Top Cover (Autodesk Fusion 360 design; units mm, degrees)
Autodesk Fusion 360 part; units mm, degrees
sketch "Sketch1" plane through (0, 0, 0) normal (0, 0, 1) x (1, 0, 0)
  line L0 (0, 0) -> (-187, 0)
  line L1 (-187, 0) -> (-187, 128)
  line L2 (-169, 146) -> (-18, 146)
  line L3 (0, 128) -> (0, 0)
  arc A0 (0, 128) -> (-18, 146) centre (-18, 128) ccw
  arc A1 (-169, 146) -> (-187, 128) centre (-169, 128) ccw
  line L4 (-185, 2) -> (-185, 126)
  line L5 (-2, 126) -> (-2, 2)
  line L6 (-185, 2) -> (-185, 0)
  line L7 (-2, 2) -> (-2, 0)
  line L8 (-169, 142) -> (-18, 142)
  arc A2 (-169, 142) -> (-185, 126) centre (-169, 126) ccw
  arc A3 (-2, 126) -> (-18, 142) centre (-18, 126) ccw
  point P0 (0, 146)
  dimension "d1" = 187
  dimension "d2" = 146
  dimension "d3" = 18
  dimension "d4" = 18
  constraint horizontal L0
  constraint vertical L1
  constraint horizontal L2
  constraint vertical L3
  constraint coincident L0.start L3.end
  constraint coincident P0 L2
  constraint coincident P0 L3
  constraint tangent L2 A0
  constraint tangent L3 A0
  constraint tangent L1 A1
  constraint tangent L2 A1
  constraint coincident L0 L6.end
  constraint perpendicular L0 L6
  constraint coincident L0 L7.end
  constraint perpendicular L0 L7
  constraint parallel L1 L4
  constraint parallel L3 L5
  measures "d1" distance of L0.start L0.end
  measures "d2" distance of L0.start P0
  measures "d3" radius of A0
  measures "d4" radius of A1
extrude "Extrude1" add sketch "Sketch1" along normal blind 4 contours L0 L4 L5 L6 L7 L8 A2 A3
extrude "Extrude2" add sketch "Sketch1" along normal blind 2 contours L0 L1 L2 L3 A0 A1 L4 L5 L6 L7 L8 A2 A3
